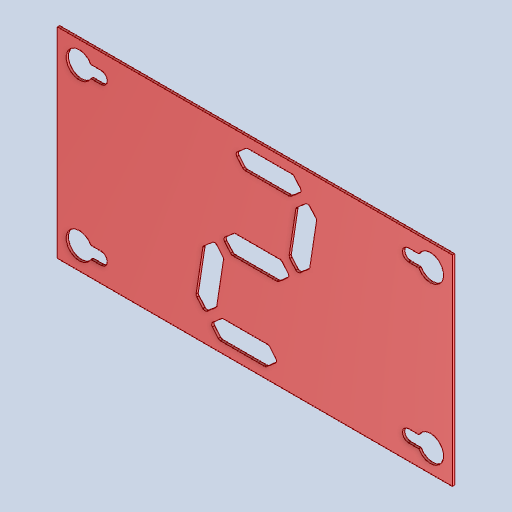
# Autodesk Inventor part: Cockpit_front_frame_cloth
Saved by Autodesk Inventor 2022.3 (Build 263350000, 350)
## iProperties
Part Number: Cockpit_front_frame_cloth
Material: PET プラスチック
Document SubType Name: Modeling
Designer: Masato Kubotera
Density: 1.541 g/cm^3
Appearance: 滑らか - 赤
Description: PP T0.75
Mass: 10.1319 g
Surface Area: 180.446 cm^2
Volume: 6.57488 cm^3
Author: Masato Kubotera
Autodesk Inventor part; units mm, degrees
ref_plane "YZ Plane" through (0, 0, 0) normal (1, 0, 0) x (0, 1, 0)
ref_plane "XZ Plane" through (0, 0, 0) normal (0, 1, 0) x (-1, 0, 0)
derived "Cockpit_front_frame.ipt"
sketch "スケッチ2" plane through (0, 0, 0) normal (0, 1, 0) x (-1, 0, 0)
  line L0 (-23.5, -22.5) -> (-28.5, -27.5)
  line L1 (-28.5, -27.5) -> (-28.5, -91)
  line L2 (-28.5, -91) -> (-23.5, -96)
  line L3 (-23.5, -96) -> (34.25, -96)
  line L4 (36.25, -98) -> (36.25, -128.5)
  line L5 (36.25, -128.5) -> (46.25, -138.5)
  line L6 (46.25, -138.5) -> (86.5, -138.5)
  line L7 (91.5, -133.5) -> (91.5, -20)
  line L8 (91.5, -20) -> (89, -17.5)
  line L9 (89, -17.5) -> (83.25, -17.5)
  line L10 (83.25, -17.5) -> (83.25, -21.0151)
  line L11 (81.7651, -22.5) -> (76.8599, -22.5)
  line L12 (75.375, -21.0151) -> (75.375, -17.5)
  line L13 (75.375, -17.5) -> (60.375, -17.5)
  line L14 (60.375, -17.5) -> (60.375, -21.0151)
  line L15 (58.8901, -22.5) -> (-23.5, -22.5)
  line L16 (-25.25, -25) -> (-20.25, -25) construction
  line L17 (-20.25, -25) -> (-20.25, -93.5) construction
  line L18 (-20.25, -93.5) -> (-25.25, -93.5) construction
  line L19 (-25.25, -93.5) -> (-25.25, -25) construction
  line L20 (-26, -25) -> (-25.25, -25) construction
  line L21 (-25.25, -93.5) -> (-26, -93.5) construction
  line L22 (-26, -93.5) -> (-26, -25) construction
  line L23 (-20.25, -93.5) -> (83.25, -93.5) construction
  line L24 (-20.25, -88.5) -> (83.25, -88.5) construction
  line L25 (83.25, -22.5) -> (83.25, -90) construction
  line L26 (83.25, -90) -> (88.25, -90) construction
  line L27 (88.25, -90) -> (88.25, -22.5) construction
  line L28 (83.25, -88.5) -> (83.25, -93.5) construction
  line L29 (83.25, -91) -> (88.25, -91) construction
  line L30 (88.25, -91) -> (88.25, -136) construction
  line L31 (83.25, -91) -> (83.25, -136) construction
  line L32 (83.25, -136) -> (88.25, -136) construction
  line L33 (38.75, -131) -> (38.75, -93.5) construction
  line L34 (43.75, -93.5) -> (43.75, -131) construction
  line L35 (38.75, -131) -> (43.75, -131) construction
  line L36 (41.25, -131) -> (41.25, -93.5) construction
  line L37 (43.75, -131) -> (81.25, -131) construction
  line L38 (81.25, -131) -> (81.25, -136) construction
  line L39 (81.25, -136) -> (43.75, -136) construction
  line L40 (43.75, -133.5) -> (81.25, -133.5) construction
  line L41 (85.75, -91) -> (85.75, -136) construction
  circle A0 centre (85.75, -133.5) radius 2.975
  arc A1 (83.25, -131) -> (88.25, -131) centre (85.75, -133.5) ccw construction
  line L42 (83.25, -91) -> (-20.25, -91) construction
  line L43 (41.25, -112.25) -> (43.75, -112.25) construction
  line L44 (62.5, -131) -> (62.5, -133.5) construction
  line L45 (41.2, -116.8151) -> (41.2, -107.6849)
  line L46 (43.8, -108.3) -> (43.8, -116.2)
  line L47 (43.8, -118.3) -> (41.2, -106.2) construction
  line L48 (41.2, -118.3) -> (43.8, -106.2) construction
  line L49 (58.55, -130.95) -> (66.45, -130.95)
  line L50 (67.0651, -133.55) -> (57.9349, -133.55)
  line L51 (56.45, -130.95) -> (68.55, -133.55) construction
  line L52 (68.55, -130.95) -> (56.45, -133.55) construction
  line L53 (41.25, -106.25) -> (43.75, -106.25) construction
  line L54 (41.25, -118.25) -> (43.75, -118.25) construction
  arc A2 (42.6849, -106.2) -> (41.2, -107.6849) centre (41.9425, -106.9425) ccw
  arc A3 (43.8, -108.3) -> (43.8, -106.2) centre (43.8, -107.25) ccw
  arc A4 (41.2, -116.8151) -> (42.6849, -118.3) centre (41.9425, -117.5575) ccw
  arc A5 (43.8, -118.3) -> (43.8, -116.2) centre (43.8, -117.25) ccw
  line L55 (56.5, -133.5) -> (56.5, -131) construction
  line L56 (68.5, -131) -> (68.5, -133.5) construction
  arc A6 (56.45, -132.0651) -> (57.9349, -133.55) centre (57.1925, -132.8075) ccw
  arc A7 (58.55, -130.95) -> (56.45, -130.95) centre (57.5, -130.95) ccw
  arc A8 (67.0651, -133.55) -> (68.55, -132.0651) centre (67.8075, -132.8075) ccw
  arc A9 (68.55, -130.95) -> (66.45, -130.95) centre (67.5, -130.95) ccw
  line L57 (56.45, -132.0651) -> (56.45, -130.95)
  line L58 (68.55, -130.95) -> (68.55, -132.0651)
  line L59 (42.6849, -106.2) -> (43.8, -106.2)
  line L60 (43.8, -118.3) -> (42.6849, -118.3)
  circle A10 centre (48.75, -133.5) radius 1.6
  line L61 (88.25, -22.5) -> (88.25, -17.5) construction
  line L62 (89, -17.5) -> (89, -90) construction
  line L63 (89, -90) -> (88.25, -90) construction
  line L64 (-13.5, -82.5) -> (-13.5, -61)
  arc A11 (-13.5, -82.5) -> (-11.5, -84.5) centre (-11.5, -82.5) ccw
  line L65 (45.5, -84.5) -> (-11.5, -84.5)
  arc A12 (45.5, -84.5) -> (47.5, -82.5) centre (45.5, -82.5) ccw
  line L66 (47.5, -61) -> (47.5, -82.5)
  arc A13 (47.5, -61) -> (45.5, -59) centre (45.5, -61) ccw
  line L67 (-11.5, -59) -> (45.5, -59)
  arc A14 (-11.5, -59) -> (-13.5, -61) centre (-11.5, -61) ccw
  line L68 (31.5, -88.5) -> (31.5, -91) construction
  line L69 (85.75, -22.5) -> (85.75, -90) construction
  circle A15 centre (85.75, -31.25) radius 1.6
  circle A16 centre (85.75, -31.25) radius 3
  circle A17 centre (85.75, -81.25) radius 1.6
  circle A18 centre (85.75, -81.25) radius 3
  line L70 (88.25, -22.5) -> (83.25, -22.5) construction
  arc A19 (88.25, -91) -> (83.25, -91) centre (85.75, -133.5) ccw construction
  circle A20 centre (48.75, -133.5) radius 3
  circle A21 centre (41.25, -98.5) radius 1.6
  circle A22 centre (41.25, -98.5) radius 3
  line L71 (10.55, -88.5) -> (10.55, -91) construction
  line L72 (52.45, -88.5) -> (52.45, -91) construction
  line L73 (51.0151, -91.05) -> (11.9849, -91.05)
  line L74 (10.5, -89.5651) -> (10.5, -88.45)
  line L75 (12.6, -88.45) -> (50.4, -88.45)
  line L76 (52.5, -88.45) -> (52.5, -89.5651)
  line L77 (52.5, -91.05) -> (10.5, -88.45) construction
  line L78 (10.5, -91.05) -> (52.5, -88.45) construction
  arc A23 (12.6, -88.45) -> (10.5, -88.45) centre (11.55, -88.45) ccw
  arc A24 (10.5, -89.5651) -> (11.9849, -91.05) centre (11.2425, -90.3075) ccw
  arc A25 (52.5, -88.45) -> (50.4, -88.45) centre (51.45, -88.45) ccw
  arc A26 (51.0151, -91.05) -> (52.5, -89.5651) centre (51.7575, -90.3075) ccw
  line L79 (-20.25, -31) -> (83.25, -31) construction
  line L80 (83.25, -26) -> (-20.25, -26) construction
  line L81 (-20.25, -26) -> (-20.25, -31) construction
  line L82 (-20.25, -28.5) -> (83.25, -28.5) construction
  line L83 (31.5, -31) -> (31.5, -26) construction
  line L84 (11.9849, -31) -> (51.0151, -31)
  arc A27 (10.5, -29.5151) -> (11.9849, -31) centre (11.2425, -30.2575) ccw
  arc A28 (51.0151, -31) -> (52.5, -29.5151) centre (51.7575, -30.2575) ccw
  line L85 (10.55, -31) -> (10.55, -26) construction
  line L86 (52.45, -26) -> (52.45, -31) construction
  circle A29 centre (6.5, -28.5) radius 1.6
  circle A30 centre (6.5, -28.5) radius 3
  line L87 (-25.25, -49.25) -> (-26, -49.25) construction
  line L88 (-25.25, -69.25) -> (-26, -69.25) construction
  line L89 (-26, -59.25) -> (-25.25, -59.25) construction
  line L90 (-22.75, -25) -> (-22.75, -93.5) construction
  arc A31 (58.8901, -22.5) -> (60.375, -21.0151) centre (59.6325, -21.7575) ccw
  arc A32 (75.375, -21.0151) -> (76.8599, -22.5) centre (76.1175, -21.7575) ccw
  line L91 (56.4375, -22.5) -> (56.4375, -17.5) construction
  line L92 (79.3125, -22.5) -> (79.3125, -17.5) construction
  circle A33 centre (-22.75, -31.75) radius 1.6
  circle A34 centre (-22.75, -31.75) radius 3
  circle A35 centre (-22.75, -86.75) radius 1.6
  circle A36 centre (-22.75, -86.75) radius 3
  line L93 (60.375, -22.5) -> (75.375, -22.5)
  line L94 (52.5, -17.5) -> (52.5, -22.5) construction
  circle A37 centre (85.75, -98.5) radius 1.475
  circle A38 centre (85.75, -103.5) radius 1.475
  circle A39 centre (85.75, -108.5) radius 1.475
  line L95 (59.5, -88.5) -> (78.75, -88.5)
  line L96 (80.75, -90.5) -> (80.75, -126.5)
  line L97 (78.75, -128.5) -> (48.25, -128.5)
  line L98 (46.25, -126.5) -> (46.25, -110)
  arc A40 (46.25, -126.5) -> (48.25, -128.5) centre (48.25, -126.5) ccw
  arc A41 (78.75, -128.5) -> (80.75, -126.5) centre (78.75, -126.5) ccw
  arc A42 (80.75, -90.5) -> (78.75, -88.5) centre (78.75, -90.5) ccw
  arc A43 (36.25, -98) -> (34.25, -96) centre (34.25, -98) ccw
  circle A44 centre (-13.5, -55) radius 1.75
  circle A45 centre (-13.5, -55) radius 2
  line L99 (23.9, -43.85) -> (10.1, -43.85) construction
  line L100 (10.1, -43.85) -> (10.1, -34.65) construction
  line L101 (10.1, -34.65) -> (23.9, -34.65) construction
  line L102 (23.9, -34.65) -> (23.9, -43.85) construction
  line L103 (23.9, -43.85) -> (10.1, -34.65) construction
  line L104 (10.1, -43.85) -> (23.9, -34.65) construction
  line L105 (9.45, -33.95) -> (24.55, -33.95) construction
  line L106 (24.55, -33.95) -> (24.55, -44.55) construction
  line L107 (24.55, -44.55) -> (9.45, -44.55) construction
  line L108 (9.45, -44.55) -> (9.45, -33.95) construction
  line L109 (9.45, -33.95) -> (24.55, -44.55) construction
  line L110 (24.55, -33.95) -> (9.45, -44.55) construction
  line L111 (10.8849, -33.9) -> (23.1151, -33.9)
  line L112 (24.6, -35.3849) -> (24.6, -43.1151)
  line L113 (24.6, -44.6) -> (9.4, -33.9) construction
  line L114 (9.4, -44.6) -> (24.6, -33.9) construction
  line L115 (23.95, -43.9) -> (10.05, -34.6) construction
  line L116 (10.05, -43.9) -> (23.95, -34.6) construction
  arc A46 (10.8849, -33.9) -> (9.4, -35.3849) centre (10.1425, -34.6425) ccw
  arc A47 (11.5349, -34.6) -> (10.05, -36.0849) centre (10.7925, -35.3425) ccw
  line L117 (9.4, -39.25) -> (24.6, -39.25) construction
  line L118 (17, -33.9) -> (17, -44.6) construction
  arc A48 (24.6, -35.3849) -> (23.1151, -33.9) centre (23.8575, -34.6425) ccw
  arc A49 (23.95, -36.0849) -> (22.4651, -34.6) centre (23.2075, -35.3425) ccw
  arc A50 (9.4, -43.1151) -> (10.8849, -44.6) centre (10.1425, -43.8575) ccw
  arc A51 (10.05, -42.4151) -> (11.5349, -43.9) centre (10.7925, -43.1575) ccw
  arc A52 (23.1151, -44.6) -> (24.6, -43.1151) centre (23.8575, -43.8575) ccw
  arc A53 (22.4651, -43.9) -> (23.95, -42.4151) centre (23.2075, -43.1575) ccw
  line L119 (11.5349, -34.6) -> (22.4651, -34.6)
  line L120 (23.95, -36.0849) -> (23.95, -42.4151)
  line L121 (9.4, -43.1151) -> (9.4, -35.3849)
  line L122 (10.05, -42.4151) -> (10.05, -36.0849)
  line L123 (22.4651, -43.9) -> (11.5349, -43.9)
  line L124 (23.1151, -44.6) -> (10.8849, -44.6)
  line L125 (-13.5, -71.75) -> (47.5, -71.75) construction
  line L126 (85.75, -56.25) -> (88.25, -56.25) construction
  line L127 (85.7, -69.2) -> (85.7, -43.3)
  line L128 (88.3049, -71.3569) -> (85.7, -41.2) construction
  line L129 (85.7, -71.3) -> (88.3, -41.2) construction
  arc A54 (85.7, -41.2) -> (85.7, -43.3) centre (85.7, -42.25) ccw
  arc A55 (88.3, -42.6849) -> (86.8151, -41.2) centre (87.5575, -41.9425) ccw
  arc A56 (85.7, -69.2) -> (85.7, -71.3) centre (85.7, -70.25) ccw
  arc A57 (86.8151, -71.3) -> (88.3, -69.8151) centre (87.5575, -70.5575) ccw
  line L130 (85.75, -41.25) -> (88.25, -41.25) construction
  line L131 (85.75, -71.25) -> (88.25, -71.25) construction
  line L132 (88.3, -42.6849) -> (88.3, -69.8151)
  line L133 (88.3, -66.8652) -> (88.3, -69.8151)
  line L134 (86.8151, -71.3) -> (85.7, -71.3)
  line L135 (85.7, -41.2) -> (86.8151, -41.2)
  line L136 (86.5, -138.5) -> (91.5, -133.5)
  arc A58 (81.7651, -22.5) -> (83.25, -21.0151) centre (82.5075, -21.7575) ccw
  circle A59 centre (85.75, -93.5) radius 2
  circle A60 centre (85.75, -93.5) radius 4 construction
  arc A61 (-13.5, -49) -> (-11.5, -51) centre (-11.5, -49) ccw construction
  line L137 (45.5, -51) -> (-11.5, -51) construction
  arc A62 (45.5, -51) -> (47.5, -49) centre (45.5, -49) ccw construction
  line L138 (10.5, -29.5151) -> (10.5, -22.5)
  line L139 (52.5, -29.5151) -> (52.5, -22.5)
  line L140 (67.875, -17.5) -> (67.875, -22.5) construction
  line L141 (52.5, -17.5) -> (83.25, -17.5) construction
  line L142 (43.75, -131) -> (43.75, -136) construction
  line L143 (57.5, -22.5) -> (57.5, -103) construction
  line L144 (57.5, -103) -> (52.5, -108) construction
  line L145 (-23.5, -108) -> (52.5, -108) construction
  line L146 (57.5, -90.5) -> (57.5, -103)
  line L147 (57.5, -103) -> (52.5, -108)
  line L148 (52.5, -108) -> (48.25, -108)
  arc A63 (59.5, -88.5) -> (57.5, -90.5) centre (59.5, -90.5) ccw
  arc A64 (48.25, -108) -> (46.25, -110) centre (48.25, -110) ccw
  circle A65 centre (56.5, -28.5) radius 1.6
  circle A66 centre (56.5, -28.5) radius 3
  line L149 (-13.5, -49) -> (-13.5, -29.5)
  point P0 (0, 0)
  point P1 (-25.7227, -96)
  point P2 (-23.5, -22.5)
  point P3 (42.5, -112.25)
  point P4 (62.5, -132.25)
  point P5 (31.5, -89.75)
  point P6 (31.5, -28.5)
  point P7 (52.5, -22)
  point P8 (46.25, -108)
  point P9 (57.5, -88.5)
  point P10 (17, -39.25)
  point P11 (17, -39.25)
  point P12 (87, -56.25)
  point P13 (17, -51)
  point P14 (10.5, -31)
  point P15 (-13.5, -39.25)
  dimension "d4" = 0.75
  measures "d4" distance of L20.start L20.end
sketch "スケッチ3" plane through (25.25, 0, 0) normal (1, 0, 0) x (0, 1, 0)
  line L0 (-135, -25) -> (0, -25)
  line L1 (0, -93.5) -> (-135, -93.5)
  line L2 (0, -25) -> (0, -93.5)
  line L3 (0, -75.7349) -> (0, -93.5)
  line L4 (-67.5, -25) -> (-67.5, -93.5) construction
  line L5 (-135, -25) -> (-135, -93.5)
  circle A0 centre (-15, -32.5) radius 2
  arc A1 (-11.4799, -34.6) -> (-11.4799, -30.4) centre (-7.5, -32.5) ccw construction
  line L6 (-7.5, -32.5) -> (-15, -32.5) construction
  arc A2 (-15, -30.4) -> (-15, -34.6) centre (-15, -32.5) ccw construction
  line L7 (-15, -30.4) -> (-11.4799, -30.4) construction
  line L8 (-15, -34.6) -> (-11.4799, -34.6) construction
  circle A3 centre (-15, -32.5) radius 3 construction
  line L9 (0, -59.25) -> (-135, -59.25) construction
  line L10 (-131, -88.5) -> (-124, -88.5)
  line L11 (-4, -88.5) -> (-4, -30)
  line L12 (-4, -30) -> (-11, -30)
  line L13 (-131, -30) -> (-131, -88.5)
  line L14 (-131, -88.5) -> (-4, -30) construction
  line L15 (-4, -88.5) -> (-131, -30) construction
  arc A4 (-11.4799, -88.1) -> (-11.4799, -83.9) centre (-7.5, -86) ccw construction
  line L16 (-15, -83.9) -> (-11.4799, -83.9) construction
  line L17 (-15, -88.1) -> (-11.4799, -88.1) construction
  arc A5 (-15, -83.9) -> (-15, -88.1) centre (-15, -86) ccw construction
  circle A6 centre (-15, -86) radius 3 construction
  circle A7 centre (-15, -86) radius 2
  arc A8 (-123.5201, -83.9) -> (-123.5201, -88.1) centre (-127.5, -86) ccw construction
  line L18 (-120, -88.1) -> (-123.5201, -88.1) construction
  circle A9 centre (-120, -86) radius 3 construction
  circle A10 centre (-120, -86) radius 2
  line L19 (-120, -83.9) -> (-123.5201, -83.9) construction
  arc A11 (-120, -88.1) -> (-120, -83.9) centre (-120, -86) ccw construction
  arc A12 (-123.5201, -30.4) -> (-123.5201, -34.6) centre (-127.5, -32.5) ccw construction
  line L20 (-120, -34.6) -> (-123.5201, -34.6) construction
  circle A13 centre (-120, -32.5) radius 3 construction
  arc A14 (-120, -34.6) -> (-120, -30.4) centre (-120, -32.5) ccw construction
  circle A15 centre (-120, -32.5) radius 2
  line L21 (-120, -30.4) -> (-123.5201, -30.4) construction
  line L22 (-11, -32.5) -> (-11, -30)
  line L23 (-19, -32.5) -> (-19, -30)
  line L24 (-19, -30) -> (-116, -30)
  line L25 (-124, -32.5) -> (-124, -30)
  arc A16 (-124, -32.5) -> (-116, -32.5) centre (-120, -32.5) ccw
  line L26 (-116, -32.5) -> (-116, -30)
  line L27 (-124, -86) -> (-124, -88.5)
  arc A17 (-116, -86) -> (-124, -86) centre (-120, -86) ccw
  line L28 (-116, -86) -> (-116, -88.5)
  line L29 (-11, -86) -> (-11, -88.5)
  line L30 (-19, -86) -> (-19, -88.5)
  arc A18 (-11, -86) -> (-19, -86) centre (-15, -86) ccw
  line L31 (-124, -30) -> (-131, -30)
  line L32 (-11, -88.5) -> (-4, -88.5)
  line L33 (-116, -88.5) -> (-19, -88.5)
  arc A19 (-19, -32.5) -> (-11, -32.5) centre (-15, -32.5) ccw
  point P0 (0, 0)
  point P1 (-135, -93.5)
  point P2 (-135, -25)
  point P3 (0, -26)
  point P4 (0, -26)
  point P5 (0, -26)
  point P6 (0, -31)
  point P7 (0, -31)
  point P8 (0, -31)
  point P9 (-67.5, -59.25)
ref_plane "作業平面1" through (25.25, -135, -25) normal (-1, 0, 0) x (0, 1, 0)
sketch "スケッチ4" plane through (25.25, -135, -25) normal (-1, 0, 0) x (0, 1, 0)
  line L0 (67.5, 0) -> (67.5, 68.5) construction
  line L1 (135, 68.5) -> (0, 68.5) projected
  line L2 (51.1141, 58.6095) -> (54.1517, 56.0021)
  line L3 (53.0682, 60.8859) -> (56.1057, 58.2784)
  line L4 (55.0145, 64.6885) -> (52.9607, 62.296)
  line L5 (49.704, 58.5021) -> (47.6502, 56.1095)
  line L6 (55.7733, 65.0372) -> (70.8617, 65.0372)
  line L7 (72.6043, 58.3859) -> (74.658, 60.7784)
  line L8 (71.513, 64.796) -> (74.5506, 62.1885)
  line L9 (56.7571, 58.0372) -> (71.8455, 58.0372)
  line L10 (54.4888, 55.3948) -> (56.7748, 40.4805)
  line L11 (56.5452, 39.6777) -> (54.4914, 37.2851)
  line L12 (53.0813, 37.1777) -> (50.0437, 39.7851)
  line L13 (47.4206, 55.3066) -> (49.7066, 40.3924)
  line L14 (50.3553, 59.2608) -> (53.84, 36.5264) construction
  line L15 (75.3094, 61.5372) -> (52.3094, 61.5372) construction
  arc A0 (51.1141, 58.6095) -> (49.704, 58.5021) centre (50.4628, 57.8507) ccw
  arc A1 (54.4888, 55.3948) -> (54.1517, 56.0021) centre (53.5003, 55.2433) ccw
  arc A2 (56.5452, 39.6777) -> (56.7748, 40.4805) centre (55.7864, 40.329) ccw
  arc A3 (53.0813, 37.1777) -> (54.4914, 37.2851) centre (53.7326, 37.9365) ccw
  arc A4 (49.7066, 40.3924) -> (50.0437, 39.7851) centre (50.695, 40.5439) ccw
  arc A5 (47.6502, 56.1095) -> (47.4206, 55.3066) centre (48.409, 55.4582) ccw
  arc A6 (71.8455, 58.0372) -> (72.6043, 58.3859) centre (71.8455, 59.0372) ccw
  arc A7 (74.658, 60.7784) -> (74.5506, 62.1885) centre (73.8992, 61.4298) ccw
  arc A8 (71.513, 64.796) -> (70.8617, 65.0372) centre (70.8617, 64.0372) ccw
  arc A9 (55.7733, 65.0372) -> (55.0145, 64.6885) centre (55.7733, 64.0372) ccw
  arc A10 (52.9607, 62.296) -> (53.0682, 60.8859) centre (53.7195, 61.6446) ccw
  arc A11 (56.1057, 58.2784) -> (56.7571, 58.0372) centre (56.7571, 59.0372) ccw
  line L16 (78.72, 58.6095) -> (81.7576, 56.0021)
  line L17 (77.3099, 58.5021) -> (75.2561, 56.1095)
  arc A12 (78.72, 58.6095) -> (77.3099, 58.5021) centre (78.0687, 57.8507) ccw
  line L18 (75.0264, 55.3066) -> (77.3125, 40.3924)
  arc A13 (75.2561, 56.1095) -> (75.0264, 55.3066) centre (76.0149, 55.4582) ccw
  arc A14 (82.0947, 55.3948) -> (81.7576, 56.0021) centre (81.1062, 55.2433) ccw
  line L19 (82.0947, 55.3948) -> (84.3807, 40.4805)
  arc A15 (84.151, 39.6777) -> (84.3807, 40.4805) centre (83.3922, 40.329) ccw
  line L20 (84.151, 39.6777) -> (82.0973, 37.2851)
  arc A16 (80.6871, 37.1777) -> (82.0973, 37.2851) centre (81.3385, 37.9365) ccw
  line L21 (80.6871, 37.1777) -> (77.6496, 39.7851)
  arc A17 (77.3125, 40.3924) -> (77.6496, 39.7851) centre (78.3009, 40.5439) ccw
  line L22 (55.2967, 31.3223) -> (58.3342, 28.7149)
  line L23 (53.8865, 31.2149) -> (51.8328, 28.8223)
  arc A18 (55.2967, 31.3223) -> (53.8865, 31.2149) centre (54.6453, 30.5635) ccw
  line L24 (51.6031, 28.0195) -> (53.8891, 13.1052)
  arc A19 (51.8328, 28.8223) -> (51.6031, 28.0195) centre (52.5915, 28.171) ccw
  arc A20 (58.6713, 28.1076) -> (58.3342, 28.7149) centre (57.6829, 27.9561) ccw
  line L25 (58.6713, 28.1076) -> (60.9573, 13.1934)
  arc A21 (60.7277, 12.3905) -> (60.9573, 13.1934) centre (59.9689, 13.0418) ccw
  line L26 (60.7277, 12.3905) -> (58.6739, 9.9979)
  arc A22 (57.2638, 9.8905) -> (58.6739, 9.9979) centre (57.9151, 10.6493) ccw
  line L27 (57.2638, 9.8905) -> (54.2262, 12.4979)
  arc A23 (53.8891, 13.1052) -> (54.2262, 12.4979) centre (54.8776, 13.2567) ccw
  line L28 (82.9025, 31.3223) -> (85.9401, 28.7149)
  line L29 (81.4924, 31.2149) -> (79.4386, 28.8223)
  arc A24 (82.9025, 31.3223) -> (81.4924, 31.2149) centre (82.2512, 30.5635) ccw
  line L30 (79.209, 28.0195) -> (81.495, 13.1052)
  arc A25 (79.4386, 28.8223) -> (79.209, 28.0195) centre (80.1974, 28.171) ccw
  arc A26 (86.2772, 28.1076) -> (85.9401, 28.7149) centre (85.2887, 27.9561) ccw
  line L31 (86.2772, 28.1076) -> (88.5632, 13.1934)
  arc A27 (88.3336, 12.3905) -> (88.5632, 13.1934) centre (87.5748, 13.0418) ccw
  line L32 (88.3336, 12.3905) -> (86.2798, 9.9979)
  arc A28 (84.8697, 9.8905) -> (86.2798, 9.9979) centre (85.521, 10.6493) ccw
  line L33 (84.8697, 9.8905) -> (81.8321, 12.4979)
  arc A29 (81.495, 13.1052) -> (81.8321, 12.4979) centre (82.4834, 13.2567) ccw
  line L34 (59.9558, 37.75) -> (75.0442, 37.75)
  arc A30 (59.9558, 37.75) -> (59.197, 37.4013) centre (59.9558, 36.75) ccw
  line L35 (59.197, 37.4013) -> (57.1432, 35.0088)
  arc A31 (57.1432, 35.0088) -> (57.2507, 33.5987) centre (57.902, 34.3574) ccw
  line L36 (57.2507, 33.5987) -> (60.2882, 30.9912)
  arc A32 (60.2882, 30.9912) -> (60.9396, 30.75) centre (60.9396, 31.75) ccw
  line L37 (60.9396, 30.75) -> (76.028, 30.75)
  arc A33 (76.028, 30.75) -> (76.7868, 31.0987) centre (76.028, 31.75) ccw
  line L38 (76.7868, 31.0987) -> (78.8406, 33.4912)
  arc A34 (78.8406, 33.4912) -> (78.7331, 34.9013) centre (78.0818, 34.1426) ccw
  line L39 (75.6955, 37.5088) -> (78.7331, 34.9013)
  arc A35 (75.6955, 37.5088) -> (75.0442, 37.75) centre (75.0442, 36.75) ccw
  line L40 (64.1383, 10.4628) -> (79.2267, 10.4628)
  arc A36 (64.1383, 10.4628) -> (63.3795, 10.1141) centre (64.1383, 9.4628) ccw
  line L41 (63.3795, 10.1141) -> (61.3258, 7.7216)
  arc A37 (61.3258, 7.7216) -> (61.4332, 6.3115) centre (62.0845, 7.0702) ccw
  line L42 (61.4332, 6.3115) -> (64.4708, 3.704)
  arc A38 (64.4708, 3.704) -> (65.1221, 3.4628) centre (65.1221, 4.4628) ccw
  line L43 (65.1221, 3.4628) -> (80.2105, 3.4628)
  arc A39 (80.2105, 3.4628) -> (80.9693, 3.8115) centre (80.2105, 4.4628) ccw
  line L44 (80.9693, 3.8115) -> (83.0231, 6.204)
  arc A40 (83.0231, 6.204) -> (82.9156, 7.6141) centre (82.2643, 6.8554) ccw
  line L45 (79.8781, 10.2216) -> (82.9156, 7.6141)
  arc A41 (79.8781, 10.2216) -> (79.2267, 10.4628) centre (79.2267, 9.4628) ccw
  line L46 (67.5, 37.75) -> (68.4838, 30.75) construction
  line L47 (135, 34.25) -> (0, 34.25) construction
  line L48 (0, 0) -> (135, 0) projected
  line L49 (0, 0) -> (0, 68.5) projected
  line L50 (135, 0) -> (135, 68.5) projected
  arc A42 (11.4799, 9.6) -> (11.4799, 5.4) centre (7.5, 7.5) ccw projected
  line L51 (15, 5.4) -> (11.4799, 5.4) projected
  line L52 (15, 9.6) -> (11.4799, 9.6) projected
  arc A43 (15, 5.4) -> (15, 9.6) centre (15, 7.5) ccw projected
  arc A44 (11.4799, 63.1) -> (11.4799, 58.9) centre (7.5, 61) ccw projected
  line L53 (15, 63.1) -> (11.4799, 63.1) projected
  line L54 (15, 58.9) -> (11.4799, 58.9) projected
  arc A45 (15, 58.9) -> (15, 63.1) centre (15, 61) ccw projected
  line L55 (120, 58.9) -> (123.5201, 58.9) projected
  arc A46 (120, 63.1) -> (120, 58.9) centre (120, 61) ccw projected
  line L56 (120, 63.1) -> (123.5201, 63.1) projected
  arc A47 (123.5201, 58.9) -> (123.5201, 63.1) centre (127.5, 61) ccw projected
  line L57 (120, 5.4) -> (123.5201, 5.4) projected
  arc A48 (120, 9.6) -> (120, 5.4) centre (120, 7.5) ccw projected
  arc A49 (123.5201, 5.4) -> (123.5201, 9.6) centre (127.5, 7.5) ccw projected
  line L58 (120, 9.6) -> (123.5201, 9.6) projected
  point P0 (135, -25)
  point P1 (135, 24.25)
  point P2 (135, 24.25)
  point P3 (135, 24.25)
  point P4 (47.3509, 55.7608)
  point P5 (54.4327, 55.7608)
  point P6 (56.3867, 58.0372)
  point P7 (55.3138, 65.0372)
  point P8 (71.232, 65.0372)
  point P9 (72.305, 58.0372)
  point P10 (56.8444, 40.0264)
  point P11 (49.7627, 40.0264)
  point P12 (77.9612, 59.2608)
  point P13 (82.0386, 55.7608)
  point P14 (74.9568, 55.7608)
  point P15 (77.3686, 40.0264)
  point P16 (84.4503, 40.0264)
  point P17 (81.4459, 36.5264)
  point P18 (54.5379, 31.9736)
  point P19 (58.6152, 28.4736)
  point P20 (51.5335, 28.4736)
  point P21 (53.9452, 12.7392)
  point P22 (61.027, 12.7392)
  point P23 (58.0226, 9.2392)
  point P24 (82.1437, 31.9736)
  point P25 (86.2211, 28.4736)
  point P26 (79.1393, 28.4736)
  point P27 (81.5511, 12.7392)
  point P28 (88.6328, 12.7392)
  point P29 (85.6284, 9.2392)
  point P30 (75.4145, 37.75)
  point P31 (59.4963, 37.75)
  point P32 (56.4919, 34.25)
  point P33 (60.5692, 30.75)
  point P34 (76.4875, 30.75)
  point P35 (79.4919, 34.25)
  point P36 (79.5971, 10.4628)
  point P37 (63.6788, 10.4628)
  point P38 (60.6744, 6.9628)
  point P39 (64.7518, 3.4628)
  point P40 (80.67, 3.4628)
  point P41 (83.6744, 6.9628)
  point P42 (135, 44.25)
  point P43 (135, 44.25)
  point P44 (135, 44.25)
  point P45 (67.9919, 34.25)
  dimension "d13" = 3
  dimension "d14" = 7
  dimension "d15" = 7
  dimension "d16" = 23
  dimension "d17" = 23
  dimension "d18" = 1
  dimension "d19" = 1
  dimension "d20" = 27.6059
  dimension "d21" = 27.6059
  dimension "d22" = 27.6059
  dimension "d27" = 8
  constraints: 92 end point, 86 point on line, 84 point on circle, 42 centre point, 24 tangent, 10 equal radius, 5 collinear, 5 parallel, 4 midpoint, 2 horizontal, 1 perpendicular, 185 other
  measures "d13" distance between parallel lines of L2 L3
  measures "d14" distance between parallel lines of L9 L6
  measures "d15" distance between parallel lines of L10 L13
  measures "d16" distance of L15.start L15.end
  measures "d17" distance of L14.start L14.end
  measures "d18" radius of A0
  measures "d19" radius of A6
  measures "d20" distance of L2.start L16.start
  measures "d21" distance of L2.start L22.start
  measures "d22" distance of L6.start L34.start
  measures "d27" angle of L46 L0
extrude "押し出し1" add sketch "スケッチ4" against normal blind 0.75 contours L50 L48 L49 L1 | L16 A14 L19 A15 L20 A16 L21 A17 L18 A13 L17 A12 | L22 A20 L25 A21 L26 A22 L27 A23 L24 A19 L23 A18
equation "\"d15\" = d14"
equation "\"d17\" = d16"
equation "\"d2\" = d4"
